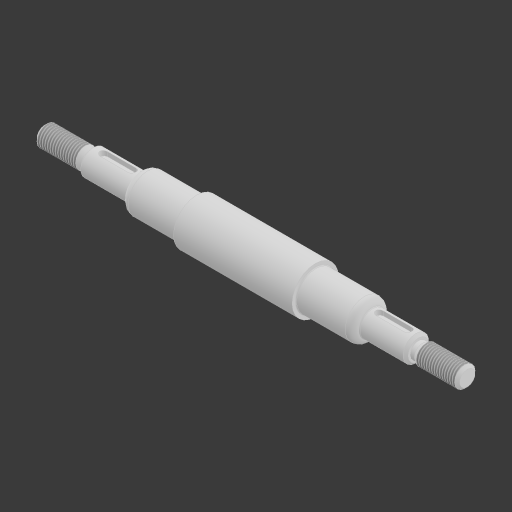
# Autodesk Inventor part: 부품1
Saved by Autodesk Inventor 2023 (Build 270158000, 158)
## iProperties
Created: 2022-11-27
Part Number: 부품1
Material: 일반
Document SubType Name: Modeling
Designer: a2474
Mass: 23.8021 g
Surface Area: 72.0757 cm^2
Volume: 23.8021 cm^3
Density: 1 g/cm^3
Appearance: 기본값
Author: a2474
Autodesk Inventor part; units mm, degrees
ref_plane "YZ Plane" through (0, 0, 0) normal (1, 0, 0) x (0, 1, 0)
sketch "스케치1" plane through (0, 0, 0) normal (0, 0, 1) x (1, 0, 0)
  line L0 (-32.6496, 0.1257) -> (-13.6496, 0.1257)
  line L1 (-13.6496, 0.1257) -> (-13.6496, 4.1257)
  line L2 (-13.6496, 4.1257) -> (-32.6496, 4.1257)
  line L3 (-32.6496, 4.1257) -> (-32.6496, 0.1257)
  line L4 (-13.6496, 0.1257) -> (4.3504, 0.1257)
  line L5 (4.3504, 0.1257) -> (4.3504, 5.1257)
  line L6 (4.3504, 5.1257) -> (-13.6496, 5.1257)
  line L7 (-13.6496, 5.1257) -> (-13.6496, 0.1257)
  line L8 (4.3504, 0.1257) -> (26.3504, 0.1257)
  line L9 (26.3504, 0.1257) -> (26.3504, 7.6257)
  line L10 (26.3504, 7.6257) -> (4.3504, 7.6257)
  line L11 (4.3504, 7.6257) -> (4.3504, 0.1257)
  line L12 (26.3504, 0.1257) -> (72.3504, 0.1257)
  line L13 (72.3504, 0.1257) -> (72.3504, 9.1257)
  line L14 (72.3504, 9.1257) -> (26.3504, 9.1257)
  line L15 (26.3504, 9.1257) -> (26.3504, 0.1257)
  line L16 (72.3504, 0.1257) -> (94.3504, 0.1257)
  line L17 (94.3504, 0.1257) -> (94.3504, 7.6257)
  line L18 (94.3504, 7.6257) -> (72.3504, 7.6257)
  line L19 (72.3504, 7.6257) -> (72.3504, 0.1257)
  line L20 (94.3504, 0.1257) -> (112.3504, 0.1257)
  line L21 (112.3504, 0.1257) -> (112.3504, 5.1257)
  line L22 (112.3504, 5.1257) -> (94.3504, 5.1257)
  line L23 (94.3504, 5.1257) -> (94.3504, 0.1257)
  line L24 (112.3504, 0.1257) -> (131.3504, 0.1257)
  line L25 (131.3504, 0.1257) -> (131.3504, 4.1257)
  line L26 (131.3504, 4.1257) -> (112.3504, 4.1257)
  line L27 (112.3504, 4.1257) -> (112.3504, 0.1257)
  dimension "d6" = 19
  dimension "d7" = 4
  dimension "d8" = 18
  dimension "d9" = 5
  dimension "d10" = 22
  dimension "d11" = 7.5
  dimension "d12" = 46
  dimension "d13" = 9
  dimension "d14" = 22
  dimension "d15" = 7.5
  dimension "d16" = 18
  dimension "d17" = 5
  dimension "d18" = 19
  dimension "d19" = 4
  constraints: 56 end point, 14 parallel, 7 horizontal, 7 perpendicular
  measures "d6" distance of L2.end L1.end
  measures "d7" distance of L1.end L0.end
  measures "d8" distance of L6.end L5.end
  measures "d9" distance of L5.end L4.end
  measures "d10" distance of L10.end L9.end
  measures "d11" distance of L9.end L8.end
  measures "d12" distance of L14.end L13.end
  measures "d13" distance of L13.end L12.end
  measures "d14" distance of L18.end L17.end
  measures "d15" distance of L17.end L16.end
  measures "d16" distance of L22.end L21.end
  measures "d17" distance of L21.end L20.end
  measures "d18" distance of L26.end L25.end
  measures "d19" distance of L25.end L24.end
revolve "회전1" add sketch "스케치1" angle 360 about axis through (4.3504, 0.1257, 0) along (1, 0, 0)
ref_plane "작업 평면1" through (0, 3.2, 0) normal (0, 1, 0) x (-1, 0, 0)
sketch "스케치2" plane through (0, 3.2, 0) normal (0, 1, 0) x (-1, 0, 0)
  line L0 (9.6496, 0) -> (-1.3504, 0) construction
  line L1 (9.6496, 1.5) -> (-1.3504, 1.5)
  line L2 (-1.3504, -1.5) -> (9.6496, -1.5)
  arc A0 (9.6496, -1.5) -> (9.6496, 1.5) centre (9.6496, 0) ccw
  arc A1 (-1.3504, 1.5) -> (-1.3504, -1.5) centre (-1.3504, 0) ccw
  line L3 (-4.3504, 5) -> (-4.3504, -5) projected
  point P0 (0, 0)
  point P1 (4.1496, 0)
  point P2 (11.1496, 0)
  point P3 (-2.8504, 0)
  dimension "d23" = 3
  dimension "d24" = 14
  dimension "d25" = 3
  constraints: 8 end point, 6 point on circle, 4 tangent, 2 centre point, 1 horizontal, 1 horizontal alignment, 1 midpoint, 1 parallel
  measures "d23" distance between parallel lines of L1 L2
  measures "d24" distance of point (11.15, 0) point (-2.85, 0)
  measures "d25" distance from line of L3 L0.end
extrude "돌출1" cut sketch "스케치2" along normal blind 10
chamfer "모따기1" distance 1 angle 45 2 edges at (131.3504, -3.8743, 0) (-32.6496, -3.8743, 0)
sketch "스케치3" plane through (0, 0, 0) normal (0, 1, 0) x (-1, 0, 0)
  line L0 (-4.3504, 5) -> (-4.3504, -5) projected
  line L1 (13.6496, 4) -> (13.6496, -4) projected
  line L2 (13.6496, -3.2) -> (15.2496, -3.2)
  line L3 (15.2496, -3.2) -> (16.6353, -4)
  line L4 (31.6496, -4) -> (13.6496, -4) projected
  line L5 (16.6859, -4) -> (13.6496, -4)
  line L6 (13.6496, -3.2) -> (13.6496, -4)
  line L7 (38.8496, 0) -> (-11.5504, 0) projected
  line L8 (16.6353, -4) -> (19.0062, -5.3688)
  line L9 (19.0062, -5.3688) -> (13.6496, -5.3688)
  line L10 (13.6496, -4) -> (13.6496, -5.3688)
  line L11 (13.6496, 5) -> (13.6496, -5) projected
  point P0 (0, 0)
  dimension "d34" = 30
  dimension "d35" = 1.6
  dimension "d36" = 0.8
  constraints: 14 end point, 3 point on line, 2 collinear, 2 horizontal, 1 perpendicular
  measures "d34" angle of L4 L3
  measures "d35" distance of L2.start L2.end
  measures "d36" distance between parallel lines of L4 L2
revolve "회전2" cut sketch "스케치3" angle 360 about axis through (-10, 0, 0) along (-1, 0, 0)
sketch "스케치4" plane through (0, 0, 0) normal (0, 0, 1) x (1, 0, 0)
  point P0 (0, 0)
ref_plane "작업 평면2" through (49.3504, 0.1257, 0) normal (1, 0, 0) x (0, 0, -1)
mirror "미러1" about plane through (49.3504, 0.1257, 0) normal (1, 0, 0) of "회전2", "돌출1"
chamfer "모따기2" distance 1 angle 45 1 edges at (112.3504, -4.8743, 0)
fillet "모깎기1" radius 0.3 4 edges at (94.3504, -4.8743, 0) (4.3504, -4.8743, 0) (26.3504, -7.3743, 0) (72.3504, -7.3743, 0)
fillet "모깎기2" radius 3 2 edges at (94.3504, -7.3743, 0) (4.3504, -7.3743, 0)
thread "스레드1" size "M8x1" class "6g" standard "ANSI Metric M Profile" full length
